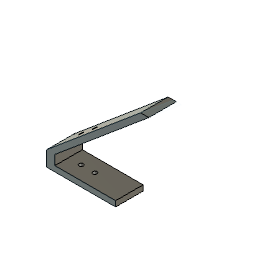
Ständer (Autodesk Fusion 360 design; units mm, degrees)
Autodesk Fusion 360 part; units mm, degrees
sketch "Skizze1" plane through (0, 0, 0) normal (0, 0, 1) x (1, 0, 0)
  line L0 (0, 0) -> (50, 0)
  line L1 (50, 0) -> (50, 20)
  line L2 (50, 20) -> (0, 20)
  line L3 (0, 20) -> (0, 0)
  line L4 (0, 20) -> (50, 0) construction
  line L5 (25, 10) -> (30, 10) construction
  line L6 (25, 10) -> (20, 10) construction
  circle A0 centre (20, 10) radius 1.5
  circle A1 centre (30, 10) radius 1.5
  dimension "d1" = 50
  dimension "d2" = 20
  dimension "d3" = 5
  dimension "d4" = 5
  dimension "d5" = 3
  dimension "d6" = 3
  constraint horizontal L0
  constraint vertical L1
  constraint horizontal L2
  constraint vertical L3
  constraint coincident L0.start L3.end
  constraint midpoint L4 L5.start
  constraint horizontal L5
  constraint parallel L5 L6
  constraint coincident L6.end A0.centre
  constraint coincident L5.end A1.centre
  measures "d1" distance of L0.start L0.end
  measures "d2" distance of L0.start L2.end
  measures "d3" distance of L5.start L5.end
  measures "d4" distance of L5.start L6.end
  measures "d5" diameter of A0
  measures "d6" diameter of A1
extrude "Extrusion1" add sketch "Skizze1" along normal blind 3
extrude "Extrusion2" add 1 faces at (43.8333, 10, 3) along direction (0, 0, 1) blind 1
sketch "Skizze2" plane through (0, 0, 0) normal (0, -1, 0) x (1, 0, 0)
  line L0 (0, 0) -> (50, 0)
  line L1 (50, 0) -> (50, 4)
  line L2 (50, 4) -> (0, 4)
  line L3 (0, 4) -> (0, 0)
  line L4 (0, 4) -> (0, 11)
  line L5 (0, 11) -> (91.9253, 88.1345)
  line L6 (0, 11) -> (120, 11) construction
  line L7 (0, 11) -> (6, 11)
  line L8 (6, 11) -> (97.9253, 88.1345)
  line L9 (6, 11) -> (126, 11) construction
  line L10 (91.9253, 88.1345) -> (97.9253, 88.1345)
  line L11 (6, 11) -> (6, 4)
  dimension "d11" = 7
  dimension "d12" = 120
  dimension "d13" = 40
  dimension "d14" = 6
  dimension "d15" = 40
  dimension "d16" = 120
  constraint coincident L2.end L3.start
  constraint perpendicular L2 L4
  constraint horizontal L6
  constraint perpendicular L4 L7
  constraint horizontal L9
  constraint coincident L2 L11.end
  constraint perpendicular L2 L11
  measures "d11" distance of L2.end L4.end
  measures "d12" distance of L4.end L5.end
  measures "d13" angle of L5 L6
  measures "d14" distance of L4.end L7.end
  measures "d15" angle of L8 L9
  measures "d16" distance of L7.end L8.end
extrude "Extrusion3" add sketch "Skizze2" against normal blind 20 contours L2 L4 L7 L11 | L5 L7 L8 L10
sketch "Skizze3" plane through (0, 0, 4) normal (0, 0, 1) x (-1, 0, 0)
  line L0 (-6, -20) -> (-6, 0)
  line L1 (-6, 0) -> (-50, 0)
  line L2 (-50, 0) -> (-50, -20)
  line L3 (-50, -20) -> (-6, -20)
  circle A0 centre (-30, -10) radius 1.5
  circle A1 centre (-20, -10) radius 1.5
extrude "Extrusion4" cut sketch "Skizze3" along normal blind 69 contours A0 | A1
sketch "Skizze4" plane through (0, 0, 0) normal (0, -1, 0) x (1, 0, 0)
  line L0 (0, 0) -> (50, 0)
  line L1 (50, 0) -> (50, 4)
  line L2 (50, 4) -> (6, 4)
  line L3 (6, 4) -> (6, 11)
  line L4 (6, 11) -> (97.9253, 88.1345)
  line L5 (97.9253, 88.1345) -> (91.9253, 88.1345)
  line L6 (91.9253, 88.1345) -> (0, 11)
  line L7 (0, 11) -> (0, 0)
move_face "Flächen versetzen1" offset -20 1 faces at (93.9253, 6.6667, 88.1345)
move_face "Fläche verschieben1" to x (1, 0, 0) y (0, 1, 0) z (0, 0, 1) at (-5, 0, 0) 2 faces at (21.4981, 10.0748, 1.3333) (31.4981, 10.0748, 1.3333)
delete_face "Fläche löschen1" 1 faces at (20.0432, 11.4994, 26.14)
delete_face "Fläche löschen2" 1 faces at (29.9887, 11.5, 32.8071)
sketch "Skizze5" plane through (-5.4164, 0, 6.4551) normal (-0.642788, 0, 0.766044) x (0, -1, 0)
  line L0 (0, 7.0707) -> (0, 95.9562)
  line L1 (0, 95.9562) -> (-20, 95.9562)
  line L2 (-20, 95.9562) -> (-20, 7.0707)
  line L3 (-20, 7.0707) -> (0, 7.0707)
sketch "Skizze6" plane through (0, 0, 4) normal (0, 0, 1) x (-1, 0, 0)
  line L0 (-6, -20) -> (-6, 0)
  line L1 (-6, 0) -> (-50, 0)
  line L2 (-50, 0) -> (-50, -20)
  line L3 (-50, -20) -> (-6, -20)
  circle A0 centre (-25, -10) radius 1.5
  circle A1 centre (-15, -10) radius 1.5
extrude "Extrusion5" cut sketch "Skizze6" along normal blind 59 contours A0 | A1
equation "d17 = 0.00 mm - 20 mm"
